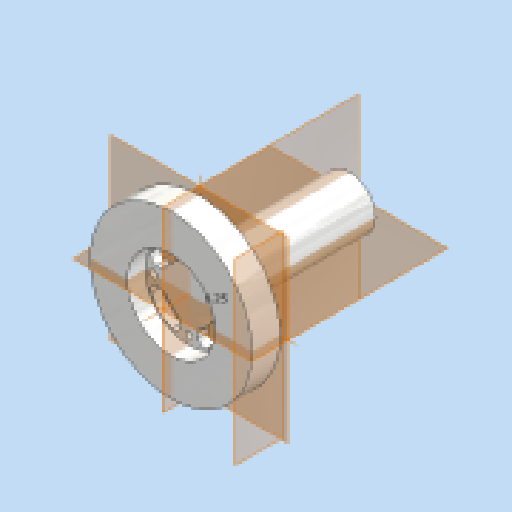
# Autodesk Inventor part: MotorHousingV2
Saved by Autodesk Inventor 2027 (Build 310192060, 192F)
## iProperties
Created: 2025-04-12
Part Number: MotorHousingV2
Material: Plastic, Opaque White
Document SubType Name: Modeling
Designer: georg
Density: 0.952 g/cm^3
Appearance: Smooth - White
Mass: 87.7582 g
Surface Area: 190.341 cm^2
Volume: 92.183 cm^3
Author: georg
Autodesk Inventor part; units mm, degrees
sketch "Sketch1" plane through (0, 0, 0) normal (0, 0, 1) x (1, 0, 0)
  circle A0 centre (0, 0) radius 40.5
  dimension "d0" = 81
  constraints: 1 centre point, 1 coincident
  measures "d0" diameter of A0
extrude "Extrusion1" add sketch "Sketch1" along normal blind 14
sketch "Sketch2" plane through (0, 0, 14) normal (0, 0, 1) x (1, 0, 0)
  circle A0 centre (0, 0) radius 22
  dimension "d3" = 44
  constraints: 1 centre point, 1 coincident
  measures "d3" diameter of A0
extrude "Extrusion2" cut sketch "Sketch2" against normal blind 9
sketch "Sketch3" plane through (0, 0, 5) normal (0, 0, 1) x (1, 0, 0)
  circle A0 centre (0, 18) radius 2
  circle A1 centre (-18, 0) radius 2
  circle A2 centre (0, -18) radius 2
  circle A3 centre (18, 0) radius 2
  point P0 (0, 0)
  dimension "d6" = 4
  dimension "d7" = 18
  dimension "d10" = 360
  constraints: 4 centre point, 9 other
  measures "d6" diameter of A0
  measures "d7" distance of point (0, 0) A0.centre
extrude "Extrusion3" cut sketch "Sketch3" against normal blind 12.75
sketch "Sketch4" plane through (0, 0, 5) normal (0, 0, 1) x (1, 0, 0)
  arc A0 (-4.5165, 17.448) -> (-8.8542, 19.2414) centre (-7.5165, 16.3345) ccw
  arc A1 (-8.8542, 19.2414) -> (-19.0977, 9.16) centre (0, 0) ccw
  arc A2 (-19.0977, 9.16) -> (-17.4931, 4.4714) centre (-16.3796, 7.4714) ccw
  arc A3 (-14.1333, 4.5) -> (-11.4833, 6.0938) centre (-14.1333, 7.5) ccw
  line L0 (-4.5, 14.1333) -> (-4.5, 16.3631)
  arc A4 (-4.5, 16.3631) -> (-8.75, 19.0902) centre (-7.5, 16.3631) ccw
  arc A5 (-6.0938, 11.4833) -> (-4.5, 14.1333) centre (-7.5, 14.1333) ccw
  arc A6 (-6.0938, 11.4833) -> (-11.4833, 6.0938) centre (0, 0) ccw
  arc A7 (-8.8542, 19.2414) -> (-19.2547, 8.8254) centre (0, 0) ccw
  arc A8 (-8.75, 19.0902) -> (-19.0902, 8.75) centre (0, 0) ccw
  arc A9 (-19.0902, 8.75) -> (-16.3631, 4.5) centre (-16.3631, 7.5) ccw
  line L1 (-16.3631, 4.5) -> (-14.1333, 4.5)
  arc A10 (-11.4833, -6.0938) -> (-14.1333, -4.5) centre (-14.1333, -7.5) ccw
  arc A11 (-4.5, -14.1333) -> (-6.0938, -11.4833) centre (-7.5, -14.1333) ccw
  arc A12 (-11.4833, -6.0938) -> (-6.0938, -11.4833) centre (0, 0) ccw
  line L2 (-14.1333, -4.5) -> (-16.3631, -4.5)
  line L3 (-4.5, -16.3631) -> (-4.5, -14.1333)
  arc A13 (-16.3631, -4.5) -> (-19.0902, -8.75) centre (-16.3631, -7.5) ccw
  arc A14 (-17.448, -4.5165) -> (-19.2414, -8.8542) centre (-16.3345, -7.5165) ccw
  arc A15 (-8.75, -19.0902) -> (-4.5, -16.3631) centre (-7.5, -16.3631) ccw
  arc A16 (-9.16, -19.0977) -> (-4.4714, -17.4931) centre (-7.4714, -16.3796) ccw
  arc A17 (-19.0902, -8.75) -> (-8.75, -19.0902) centre (0, 0) ccw
  arc A18 (-19.2414, -8.8542) -> (-9.16, -19.0977) centre (0, 0) ccw
  arc A19 (-19.2414, -8.8542) -> (-8.8254, -19.2547) centre (0, 0) ccw
  arc A20 (6.0938, -11.4833) -> (4.5, -14.1333) centre (7.5, -14.1333) ccw
  arc A21 (14.1333, -4.5) -> (11.4833, -6.0938) centre (14.1333, -7.5) ccw
  arc A22 (6.0938, -11.4833) -> (11.4833, -6.0938) centre (0, 0) ccw
  line L4 (4.5, -14.1333) -> (4.5, -16.3631)
  line L5 (16.3631, -4.5) -> (14.1333, -4.5)
  arc A23 (4.5, -16.3631) -> (8.75, -19.0902) centre (7.5, -16.3631) ccw
  arc A24 (4.5165, -17.448) -> (8.8542, -19.2414) centre (7.5165, -16.3345) ccw
  arc A25 (19.0902, -8.75) -> (16.3631, -4.5) centre (16.3631, -7.5) ccw
  arc A26 (19.0977, -9.16) -> (17.4931, -4.4714) centre (16.3796, -7.4714) ccw
  arc A27 (8.75, -19.0902) -> (19.0902, -8.75) centre (0, 0) ccw
  arc A28 (8.8542, -19.2414) -> (19.0977, -9.16) centre (0, 0) ccw
  arc A29 (8.8542, -19.2414) -> (19.2547, -8.8254) centre (0, 0) ccw
  arc A30 (11.4833, 6.0938) -> (14.1333, 4.5) centre (14.1333, 7.5) ccw
  arc A31 (4.5, 14.1333) -> (6.0938, 11.4833) centre (7.5, 14.1333) ccw
  arc A32 (11.4833, 6.0938) -> (6.0938, 11.4833) centre (0, 0) ccw
  line L6 (14.1333, 4.5) -> (16.3631, 4.5)
  line L7 (4.5, 16.3631) -> (4.5, 14.1333)
  arc A33 (16.3631, 4.5) -> (19.0902, 8.75) centre (16.3631, 7.5) ccw
  arc A34 (17.448, 4.5165) -> (19.2414, 8.8542) centre (16.3345, 7.5165) ccw
  arc A35 (8.75, 19.0902) -> (4.5, 16.3631) centre (7.5, 16.3631) ccw
  arc A36 (9.16, 19.0977) -> (4.4714, 17.4931) centre (7.4714, 16.3796) ccw
  arc A37 (19.0902, 8.75) -> (8.75, 19.0902) centre (0, 0) ccw
  arc A38 (19.2414, 8.8542) -> (9.16, 19.0977) centre (0, 0) ccw
  arc A39 (19.2414, 8.8542) -> (8.8254, 19.2547) centre (0, 0) ccw
  point P0 (41.0732, 32.7294)
  dimension "d16" = 360
  constraints: 72 point on circle, 36 centre point, 16 end point, 6 coincident, 157 other
extrude "Extrusion4" cut sketch "Sketch4" against normal blind 12.75
ref_plane "Work Plane1" through (40.7, 0, 0) normal (1, 0, 0) x (0, 1, 0)
sketch "Sketch7" plane through (0, 0, 0) normal (0, 0, -1) x (-1, 0, 0)
  circle A0 centre (0, 0) radius 10
  circle A1 centre (0, 0) radius 5
  circle A2 centre (0, 0) radius 13
  arc A3 (-14.1333, 4.5) -> (-11.4833, 6.0938) centre (-14.1333, 7.5) ccw projected
  circle A4 centre (0, 0) radius 10.25
  point P0 (0, 0)
  dimension "d32" = 0.25
  constraints: 3 centre point, 1 coincident, 7 other
  measures "d32" radial gap between concentric circles of A0 A4
extrude "Extrusion6" add sketch "Sketch7" along normal blind 75.2375 contours A2
extrude "Extrusion7" add sketch "Sketch7" along normal blind 70 contours A0 | A1
sketch "Sketch8" plane through (0, 0, -70) normal (0, 0, -1) x (-1, 0, 0)
  line L0 (0, 6.6395) -> (5.75, 3.3198)
  line L1 (5.75, 3.3198) -> (5.75, -3.3198)
  line L2 (5.75, -3.3198) -> (0, -6.6395)
  line L3 (0, -6.6395) -> (-5.75, -3.3198)
  line L4 (-5.75, -3.3198) -> (-5.75, 3.3198)
  line L5 (-5.75, 3.3198) -> (0, 6.6395)
  point P0 (0, 0)
  point P1 (0, 0)
  constraints: 12 end point, 1 coincident, 13 other
extrude "Extrusion8" cut sketch "Sketch8" against normal blind 10
body "Solid1"
